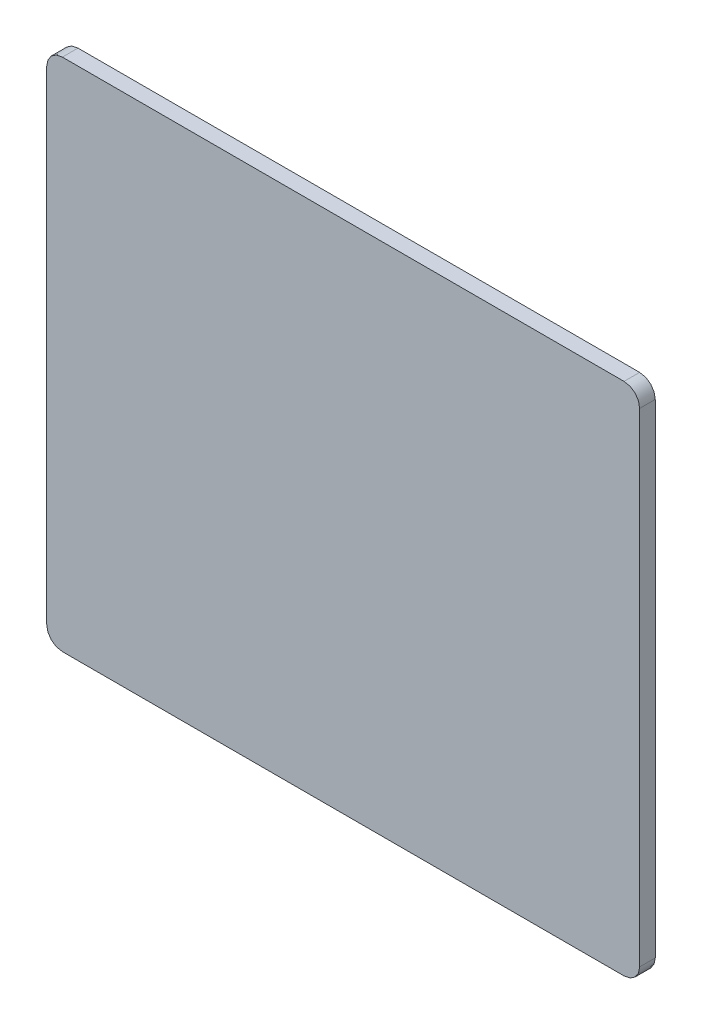
# Autodesk Inventor part: Sitzfläche_Glas
Saved by Autodesk Inventor 2018.2 (Build 222227000, 227)
## iProperties
Created: 2019-03-20
Part Number: Sitzfläche_Glas
Material: Glas
Document SubType Name: Modeling
Designer: Lolob
Density: 2.18 g/cm^3
Appearance: Klar
Author: Lolob
Autodesk Inventor part; units mm, degrees
ref_plane "YZ Plane" through (0, 0, 0) normal (1, 0, 0) x (0, 1, 0)
ref_plane "XZ Plane" through (0, 0, 0) normal (0, 1, 0) x (-1, 0, 0)
ref_plane "XY Plane" through (0, 0, 0) normal (0, 0, 1) x (1, 0, 0)
ref_plane "Arbeitsebene2" through (0, 0, 0) normal (0, 0, 1) x (1, 0, 0)
sketch "Skizze2" plane through (0, 0, 0) normal (0, 0, 1) x (1, 0, 0)
  arc A0 (170, -155) -> (180, -145) centre (170, -145) ccw projected
  line L0 (-170, -155) -> (170, -155) projected
  arc A1 (-180, -145) -> (-170, -155) centre (-170, -145) ccw projected
  line L1 (-180, 145) -> (-180, -145) projected
  arc A2 (-170, 155) -> (-180, 145) centre (-170, 145) ccw projected
  line L2 (170, 155) -> (-170, 155) projected
  arc A3 (180, 145) -> (170, 155) centre (170, 145) ccw projected
  line L3 (180, -145) -> (180, 145) projected
  line L4 (190, -155) -> (190, 155) projected
  arc A4 (190, 155) -> (180, 165) centre (180, 155) ccw projected
  line L5 (180, 165) -> (-180, 165) projected
  arc A5 (-180, 165) -> (-190, 155) centre (-180, 155) ccw projected
  line L6 (-190, -155) -> (-190, 155) projected
  arc A6 (-190, -155) -> (-180, -165) centre (-180, -155) ccw projected
  line L7 (-180, -165) -> (180, -165) projected
  arc A7 (180, -165) -> (190, -155) centre (180, -155) ccw projected
  line L8 (190, 155) -> (190, -155)
  line L9 (180, -165) -> (-180, -165)
  line L10 (-190, -155) -> (-190, 155)
  line L11 (-180, 165) -> (180, 165)
  arc A8 (190, 155) -> (180, 165) centre (180, 155) ccw
  arc A9 (180, -165) -> (190, -155) centre (180, -155) ccw
  arc A10 (-190, -155) -> (-180, -165) centre (-180, -155) ccw
  arc A11 (-180, 165) -> (-190, 155) centre (-180, 155) ccw
  point P0 (0, 0)
  constraints: 9 point on circle, 8 end point, 4 centre point, 2 collinear, 2 concentric, 2 tangent, 1 vertical
extrude "Extrusion1" add sketch "Skizze2" along normal blind 10 contours L0 A1 L1 A2 L2 A3 L3 A0 | A7 L7 A6 L6 A5 L5 A4 L4
